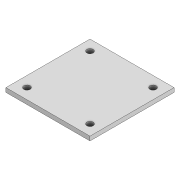
# Autodesk Inventor part: vertical batter holder 4 holes in bottom drill template
Saved by Autodesk Inventor 2020 (Build 240168000, 168)
## iProperties
Created: 2020-01-30
Part Number: vertical batter holder 4 holes in bottom drill template
Material: Generic
Document SubType Name: Modeling
Designer: ball
Density: 1 g/cm^3
Appearance: Default
Author: ball
Autodesk Inventor part; units mm, degrees
ref_plane "YZ Plane" through (0, 0, 0) normal (1, 0, 0) x (0, 1, 0)
ref_plane "XZ Plane" through (0, 0, 0) normal (0, 1, 0) x (-1, 0, 0)
ref_plane "XY Plane" through (0, 0, 0) normal (0, 0, 1) x (1, 0, 0)
sketch "Sketch1" plane through (0, 0, 0) normal (0, 1, 0) x (-1, 0, 0)
  line L0 (25.4, 25.4) -> (-25.4, 25.4)
  line L1 (-25.4, 25.4) -> (-25.4, -25.4)
  line L2 (-25.4, -25.4) -> (25.4, -25.4)
  line L3 (25.4, -25.4) -> (25.4, 25.4)
  line L4 (25.4, 25.4) -> (-25.4, -25.4) construction
  line L5 (-25.4, 25.4) -> (25.4, -25.4) construction
  point P0 (0, 0)
  dimension "d0" = 50.8
  dimension "d1" = 50.8
  constraints: 12 end point, 2 midpoint, 2 parallel, 1 horizontal, 1 perpendicular
  measures "d0" distance of L2.end L1.end
  measures "d1" distance of L1.end L0.end
extrude "Extrusion1" add sketch "Sketch1" along normal blind 2.54
sketch "Sketch2" plane through (0, 2.54, 0) normal (0, 1, 0) x (1, 0, 0)
  line L0 (-25.4, -25.4) -> (25.4, -25.4) projected
  line L1 (-25.4, 25.4) -> (-25.4, -25.4) projected
  line L2 (25.4, -25.4) -> (25.4, 25.4) projected
  line L3 (25.4, 25.4) -> (-25.4, 25.4) projected
  point P0 (0, 0)
  point P1 (-19.05, -19.05)
  point P2 (-19.05, 19.05)
  point P3 (19.05, 19.05)
  point P4 (19.05, -19.05)
  dimension "d4" = 6.35
  dimension "d5" = 6.35
  dimension "d6" = 6.35
  dimension "d7" = 6.35
  dimension "d8" = 6.35
  dimension "d9" = 6.35
  dimension "d10" = 6.35
  dimension "d11" = 6.35
  measures "d4" distance from line of L0 point (-19.05, -19.05)
  measures "d5" distance from line of L1 point (-19.05, -19.05)
  measures "d6" distance from line of L2 point (19.05, -19.05)
  measures "d7" distance from line of L0 point (19.05, -19.05)
  measures "d8" distance from line of L2 point (19.05, 19.05)
  measures "d9" distance from line of L3 point (19.05, 19.05)
  measures "d10" distance from line of L3 point (-19.05, 19.05)
  measures "d11" distance from line of L1 point (-19.05, 19.05)
hole "Hole1" at (-19.05, 2.54, 19.05) at (19.05, 2.54, 19.05) at (19.05, 2.54, -19.05) at (-19.05, 2.54, -19.05) direction (0, -1, 0) diameter 3.8608 end through all
equation "\"d6\" = d5"
equation "\"d7\" = d4"
equation "\"d8\" = d6"
equation "\"d9\" = d4"
equation "\"d10\" = d4"
equation "\"d11\" = d5"
body "Solid1"
